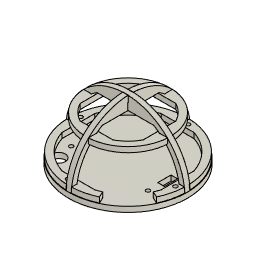
Ball prototype (Autodesk Fusion 360 design; units mm, degrees)
Autodesk Fusion 360 part; units mm, degrees
sketch "Schizzo2" plane through (0, 0, 0) normal (1, 0, 0) x (0, 1, 0)
  circle A0 centre (0, 0) radius 45 construction
  line L0 (0, -45) -> (0, -43.7069)
  line L1 (0, -43.7069) -> (0, 45)
  line L2 (0, 0) -> (44.9555, 0) construction
  line L3 (44.9555, 0) -> (44.9555, 2)
  line L4 (44.9555, 0) -> (44.9555, -2)
  line L5 (0, 0) -> (-44.9555, 0) construction
  line L6 (44.9555, 2) -> (-44.9555, 2)
  line L7 (-44.9555, 2) -> (-44.9555, 0)
  line L8 (44.9555, -2) -> (-44.9555, -2)
  line L9 (-44.9555, 0) -> (-44.9555, -2)
  line L10 (44.5982, 6) -> (44.5982, 2)
  line L11 (44.5982, 6) -> (-44.5982, 6)
  line L12 (-44.5982, 6) -> (-44.5982, 2)
  arc A1 (44.9555, 2) -> (-44.9555, 2) centre (0, 0) ccw
  arc A2 (40.9512, 2) -> (-40.9512, 2) centre (0, 0) ccw
  line L13 (2, 44.9555) -> (2, 34.9555)
  line L14 (-2, 44.9555) -> (-2, 34.9555)
  line L15 (-2, 34.9555) -> (-21.4269, 34.9555)
  line L16 (2, 34.9555) -> (21.4269, 34.9555)
  line L17 (2, 34.9555) -> (-2, 34.9555)
  line L18 (2, 39.9555) -> (-2, 39.9555)
  line L19 (1.8, 39.9555) -> (1.8, 34.9555)
  line L20 (-1.8, 39.9555) -> (-1.8, 34.9555)
  line L21 (1.8, 39.9555) -> (1.8, 44.964)
  line L22 (-1.8, 39.9555) -> (-1.8, 44.964)
  line L23 (0, 0) -> (31.8198, 31.8198) construction
  line L24 (31.8198, 31.8198) -> (-31.8198, 31.8198)
  line L25 (-31.8198, 31.8198) -> (-31.8198, 27.8198)
  line L26 (-31.8198, 27.8198) -> (31.8198, 27.8198)
  line L27 (31.8198, 27.8198) -> (31.8198, 31.8198)
  line L28 (25.8554, 31.8198) -> (25.8554, 27.8198)
  line L29 (-25.8554, 31.8198) -> (-25.8554, 27.8198)
  dimension "d3" = 90
  dimension "d5" = 4
  dimension "d6" = 4
  dimension "d9" = 10
  dimension "d10" = 4
  dimension "d11" = 4
  dimension "d18" = 0.2
  dimension "d19" = 0.2
  dimension "d39" = 45
  dimension "d40" = 4
  constraint coincident A0.centre L2.start
  constraint coincident A0 L0.start
  constraint coincident A0.centre L0
  constraint coincident A0 L1.end
  constraint coincident A0.centre L1
  constraint vertical L1
  constraint perpendicular L1 L2
  constraint coincident A0 L3.end
  constraint perpendicular L2 L3
  constraint coincident A0 L4.end
  constraint perpendicular L2 L4
  constraint perpendicular L1 L5
  constraint coincident A0 L6.end
  constraint perpendicular L3 L6
  constraint coincident A0 L8.end
  constraint perpendicular L4 L8
  constraint perpendicular L5 L7
  constraint coincident A0 L10.start
  constraint coincident L6 L10.end
  constraint perpendicular L6 L10
  constraint coincident A0 L11.end
  constraint perpendicular L10 L11
  constraint coincident L6 L12.end
  constraint perpendicular L6 L12
  constraint coincident L6 A2.end
  constraint coincident L6 A2.start
  constraint vertical L13
  constraint coincident A2 L15.end
  constraint perpendicular L14 L15
  constraint coincident A2 L16.end
  constraint perpendicular L13 L16
  constraint collinear L15 L16
  constraint coincident A0 L13.start
  constraint coincident A1 L14.start
  constraint equal L13 L14
  constraint midpoint L13 L18.start
  constraint midpoint L14 L18.end
  constraint coincident L18 L19.start
  constraint coincident L17 L19.end
  constraint perpendicular L17 L19
  constraint coincident L18 L20.start
  constraint coincident L17 L20.end
  constraint perpendicular L17 L20
  constraint coincident A0 L21.end
  constraint coincident A0 L22.end
  constraint perpendicular L18 L21
  constraint perpendicular L18 L22
  constraint coincident A1 L23.end
  constraint horizontal L24
  constraint vertical L25
  constraint horizontal L26
  constraint vertical L27
  constraint coincident A1 L24.end
  constraint coincident A2 L28.start
  constraint coincident L24 L28.start
  constraint coincident L26 L28.end
  constraint perpendicular L26 L28
  constraint coincident A2 L29.start
  constraint coincident L24 L29.start
  constraint coincident L26 L29.end
  constraint perpendicular L26 L29
  measures "d3" diameter of A0
  measures "d5" distance of L6 L8
  measures "d6" distance of L11.end L12.end
  measures "d9" distance of L13.start L13.end
  measures "d10" distance of L18.start L18.end
  measures "d11" distance of A0 A2
  measures "d18" distance of L14 L20
  measures "d19" distance of L13 L19
  measures "d39" angle of L1 L23
  measures "d40" distance of L24.end L25.end
revolve "Rivoluzione1" add sketch "Schizzo2" angle 360 about axis through (0, 0, -43.7069) along (0, 0, 1) contours L1 L6 L7 L8 L9 makes body 1
revolve "Rivoluzione2" add sketch "Schizzo2" angle 360 about axis through (0, 0, -43.7069) along (0, 0, 1) separate body contours L1 L6 L11 A2 | L6 L11 L12 A2 picked at (-13.5195, 4.6667) makes body 2
revolve "Rivoluzione3" add sketch "Schizzo2" angle 360 about axis through (0, 0, -43.7069) along (0, 0, 1) separate body contours L1 L24 L26 L29 | A2 L26 L29 | A2 L24 L25 L26 makes body 3
extrude "Estrusione1" add sketch "Schizzo2" along normal mid plane 4 separate body contours L6 L10 L11 A2 | L6 L11 L12 A2 | L11 A1 A2 L26 L27 | L11 A1 A2 L25 L26 | L6 L10 A1 | L6 L12 A1 | A2 L26 L29 | A2 L26 L28 | A2 L24 L26 L27 | A2 L24 L25 L26 | A1 A2 L13 L24 | A1 A2 L14 L24 | L1 A2 L18 L22 | L1 A2 L18 L21 | L13 L17 L18 L19 | L14 L17 L18 L20 | A2 L13 L16 | A2 L14 L15 | A1 A2 L13 L21 | A1 A2 L14 L22 | L1 A1 A2 L22 | L1 A1 A2 L21 | A2 L13 L18 L21 | A2 L14 L18 L22 makes body 4
extrude "Estrusione2" add sketch "Schizzo2" along normal mid plane 4 separate body contours L6 L10 L11 A2 | L6 L11 L12 A2 | L11 A1 A2 L26 L27 | L11 A1 A2 L25 L26 | L6 L10 A1 | L6 L12 A1 | A2 L26 L29 | A2 L26 L28 | A2 L24 L26 L27 | A2 L24 L25 L26 | L1 L17 L18 L20 | L1 L17 L18 L19 | A1 A2 L13 L24 | A1 A2 L14 L24 | L13 L17 L18 L19 | L14 L17 L18 L20 | A2 L13 L16 | A2 L14 L15 | A1 A2 L13 L21 | A1 A2 L14 L22 | A2 L13 L18 L21 | A2 L14 L18 L22 makes body 5
sketch "Schizzo3" plane through (0, 0, 6) normal (0, 0, 1) x (-1, 0, 0)
  circle A0 centre (0, 0) radius 44.5982
  circle A1 centre (0, 0) radius 35.5
  circle A2 centre (0, 0) radius 37.5
  line L0 (0, 0) -> (44.5982, 0) construction
  line L1 (40.3982, 0) -> (40.3982, -1.8)
  line L2 (40.3982, -1.8) -> (44.5619, -1.8)
  line L3 (40.3982, 0) -> (40.3982, 1.8)
  line L4 (40.3982, 1.8) -> (44.5619, 1.8)
  circle A3 centre (0, 0) radius 39.5
  line L5 (37.5, 0) -> (37.5, 12.4097)
  line L6 (37.5, 0) -> (37.5, -12.4097)
  line L7 (1.8, 40.3982) -> (1.8, 44.5619)
  line L8 (0, 40.3982) -> (1.8, 40.3982)
  line L9 (-1.8, 40.3982) -> (-1.8, 44.5619)
  line L10 (0, 40.3982) -> (-1.8, 40.3982)
  line L11 (0, 37.5) -> (12.4097, 37.5)
  line L12 (0, 37.5) -> (-12.4097, 37.5)
  line L13 (-40.3982, 1.8) -> (-44.5619, 1.8)
  line L14 (-40.3982, 0) -> (-40.3982, 1.8)
  line L15 (-40.3982, -1.8) -> (-44.5619, -1.8)
  line L16 (-40.3982, 0) -> (-40.3982, -1.8)
  line L17 (-37.5, 0) -> (-37.5, 12.4097)
  line L18 (-37.5, 0) -> (-37.5, -12.4097)
  line L19 (-1.8, -40.3982) -> (-1.8, -44.5619)
  line L20 (0, -40.3982) -> (-1.8, -40.3982)
  line L21 (1.8, -40.3982) -> (1.8, -44.5619)
  line L22 (0, -40.3982) -> (1.8, -40.3982)
  line L23 (0, -37.5) -> (-12.4097, -37.5)
  line L24 (0, -37.5) -> (12.4097, -37.5)
  circle A4 centre (40.5982, -4.8) radius 1.5
  circle A5 centre (4.8, 40.5982) radius 1.5
  circle A6 centre (-40.5982, 4.8) radius 1.5
  circle A7 centre (-4.8, -40.5982) radius 1.5
  line L25 (0, 0) -> (-31.5357, 31.5357) construction
  line L26 (0, 0) -> (-40.4197, 18.848)
  line L27 (0, 0) -> (-18.848, 40.4197)
  dimension "d22" = 71
  dimension "d23" = 2
  dimension "d26" = 4.2
  dimension "d27" = 3.6
  dimension "d28" = 4
  dimension "d30" = 360
  dimension "d33" = 3
  dimension "d34" = 3
  dimension "d35" = 0.2
  dimension "d36" = 135
  dimension "d37" = 20
  dimension "d38" = 20
  constraint concentric A0 A1
  constraint concentric A1 A2
  constraint coincident A0.centre A1.centre
  constraint coincident A0 L0.end
  constraint horizontal L0
  constraint coincident L0 L1.start
  constraint perpendicular L0 L1
  constraint coincident A0 L2.end
  constraint perpendicular L0 L3
  constraint equal L1 L3
  constraint coincident A0 L4.end
  constraint perpendicular L1 L2
  constraint perpendicular L3 L4
  constraint concentric A2 A3
  constraint coincident A2 L5.start
  constraint coincident L0 L5.start
  constraint coincident A3 L5.end
  constraint tangent A2 L5
  constraint coincident A3 L6.end
  constraint tangent A2 L6
  constraint coincident A0 L25.end
  constraint coincident A0 L26.end
  constraint coincident A0 L27.end
  measures "d22" diameter of A1
  measures "d23" distance of A1 A2
  measures "d26" distance of L0.end L1
  measures "d27" distance of L2 L4
  measures "d28" distance of A1 A3
  measures "d33" diameter of A4
  measures "d34" distance of L2 A4.centre
  measures "d35" distance of L1 A4.centre
  measures "d36" angle of L0 L25
  measures "d37" angle of L25 L26
  measures "d38" angle of L25 L27
extrude "Estrusione3" cut sketch "Schizzo3" against normal blind 4 contours A0 L1 L2 L3 L4 | A0 L7 L8 L9 L10 | A0 L19 L20 L21 L22 | A0 A3 L26 L27 | A0 L13 L14 L15 L16 | A2 A3 L26 L27 | A2 A3 L12 L27 | A2 A3 L17 L26 | A1 A2 L26 L27 | A1 A2 L26 L27 | A3 A5 | A3 A5 | A2 A3 L5 L11 | A1 L26 L27 | A1 L26 L27 | A3 A6 | A3 A6 | A2 A3 L18 L23 | A2 A3 L6 L24 | A3 A4 | A3 A4 | A3 A7 | A3 A7 bodies 2
sketch "Schizzo4" plane through (0, 0, 31.8198) normal (0, 0, 1) x (-1, 0, 0)
  circle A0 centre (0, 0) radius 31.8198
  line L0 (0, 31.8198) -> (0, -31.8198) construction
  circle A1 centre (0, 0) radius 23.8198
  circle A2 centre (0, 0) radius 26.8198
  line L1 (0, -23.8198) -> (12.3255, -23.8198)
  line L2 (0, -23.8198) -> (-12.3255, -23.8198)
  line L3 (2, -25.8554) -> (-2, -25.8554)
  line L4 (-2, -25.8554) -> (-2, -30.1174)
  line L5 (2, -30.1174) -> (2, -25.8554)
  line L6 (1.8, -31.7689) -> (1.8, -26.0554)
  line L7 (1.8, -26.0554) -> (-1.8, -26.0554)
  line L8 (-1.8, -26.0554) -> (-1.8, -31.7689)
  line L9 (26.0554, -1.8) -> (31.7689, -1.8)
  line L10 (26.0554, 1.8) -> (26.0554, -1.8)
  line L11 (31.7689, 1.8) -> (26.0554, 1.8)
  line L12 (23.8198, 0) -> (23.8198, 12.3255)
  line L13 (23.8198, 0) -> (23.8198, -12.3255)
  line L14 (1.8, 26.0554) -> (1.8, 31.7689)
  line L15 (-1.8, 26.0554) -> (1.8, 26.0554)
  line L16 (-1.8, 31.7689) -> (-1.8, 26.0554)
  line L17 (0, 23.8198) -> (-12.3255, 23.8198)
  line L18 (0, 23.8198) -> (12.3255, 23.8198)
  line L19 (-26.0554, 1.8) -> (-31.7689, 1.8)
  line L20 (-26.0554, -1.8) -> (-26.0554, 1.8)
  line L21 (-31.7689, -1.8) -> (-26.0554, -1.8)
  line L22 (-23.8198, 0) -> (-23.8198, -12.3255)
  line L23 (-23.8198, 0) -> (-23.8198, 12.3255)
  point P0 (0, 31.8198)
  dimension "d44" = 5
  dimension "d45" = 8
  dimension "d62" = 0.2
  dimension "d63" = 0.2
  dimension "d64" = 0.2
  dimension "d66" = 360
  constraint coincident P0 L0.start
  constraint coincident A0 L0.end
  constraint vertical L0
  constraint concentric A0 A1
  constraint concentric A1 A2
  constraint coincident L0 L1.start
  constraint coincident A1 L1.start
  constraint coincident A2 L1.end
  constraint tangent A1 L1
  constraint coincident A2 L2.end
  constraint tangent A1 L2
  constraint coincident A0 L6.start
  constraint parallel L5 L6
  constraint perpendicular L5 L7
  constraint coincident A0 L8.end
  constraint perpendicular L7 L8
  measures "d44" distance of A0 A2
  measures "d45" distance of A0 A1
  measures "d62" distance of L5 L6
  measures "d63" distance of L4 L8
  measures "d64" distance of L3 L7
extrude "Estrusione4" cut sketch "Schizzo4" against normal blind 4 contours A0 A2 L9 L11 | A0 A2 L14 L16 | A2 L9 L10 L11 | A0 A2 L6 L8 | A2 L14 L15 L16 | A1 A2 L12 L18 | A2 L6 L7 L8 | A1 A2 L1 L13 | A0 A2 L19 L21 | A1 | A2 L19 L20 L21 | A1 A2 L17 L23 | A1 A2 L2 L22 bodies 3
sketch "Schizzo5" plane through (0, 0, 2) normal (0, 0, 1) x (-1, 0, 0)
  circle A0 centre (0, 0) radius 44.9555
  circle A1 centre (0, 0) radius 35.5 construction
  circle A2 centre (29, 13.8789) radius 1.5
  circle A3 centre (-29, 13.8789) radius 1.5
  line L0 (0, 0) -> (0, 35.5) construction
  line L1 (-29, 13.8789) -> (0, 13.8789) construction
  line L2 (0, 13.8789) -> (29, 13.8789) construction
  line L3 (-29, 13.8789) -> (0, 0) construction
  line L4 (-29, 13.8789) -> (-32.0218, 15.325) construction
  circle A4 centre (40.5982, -4.8) radius 1.5
  circle A5 centre (-40.5982, 4.8) radius 1.5
  circle A6 centre (4.8, 40.5982) radius 1.5
  circle A7 centre (-4.8, -40.5982) radius 1.5
  line L5 (0, 0) -> (-30, 0) construction
  line L6 (0, 0) -> (30, 0) construction
  line L7 (27.5, -5) -> (32.5, -5)
  line L8 (32.5, -5) -> (32.5, 5)
  line L9 (32.5, 5) -> (27.5, 5)
  line L10 (27.5, 5) -> (27.5, -5)
  line L11 (27.5, -5) -> (32.5, 5) construction
  line L12 (32.5, -5) -> (27.5, 5) construction
  line L13 (-27.5, -5) -> (-32.5, -5)
  line L14 (-32.5, -5) -> (-32.5, 5)
  line L15 (-32.5, 5) -> (-27.5, 5)
  line L16 (-27.5, 5) -> (-27.5, -5)
  line L17 (-27.5, -5) -> (-32.5, 5) construction
  line L18 (-32.5, -5) -> (-27.5, 5) construction
  line L19 (0, 0) -> (31.7884, 31.7884) construction
  circle A8 centre (26.163, 26.163) radius 5
  point P0 (30, 0)
  point P1 (-30, 0)
  dimension "d50" = 71
  dimension "d51" = 3
  dimension "d52" = 58
  dimension "d53" = 3.35
  dimension "d56" = 10
  dimension "d57" = 5
  dimension "d58" = 60
  dimension "d59" = 45
  dimension "d60" = 10
  dimension "d61" = 37
  constraint coincident A0.centre A1.centre
  constraint coincident A1 L0.end
  constraint vertical L0
  constraint coincident A3.centre L1.start
  constraint coincident L0 L1.end
  constraint perpendicular L0 L1
  constraint coincident A2.centre L2.end
  constraint perpendicular L0 L2
  constraint equal L1 L2
  constraint coincident A1 L4.end
  constraint parallel L3 L4
  constraint equal A2 A3
  constraint perpendicular L0 L5
  constraint perpendicular L0 L6
  constraint horizontal L7
  constraint perpendicular L7 L8
  constraint parallel L7 L9
  constraint parallel L8 L10
  constraint coincident L11 P0
  constraint coincident L12 P0
  constraint coincident P0 L6.end
  constraint horizontal L13
  constraint perpendicular L13 L14
  constraint parallel L13 L15
  constraint parallel L14 L16
  constraint coincident L17 P1
  constraint coincident L18 P1
  constraint coincident P1 L5.end
  constraint equal L7 L13
  constraint equal L10 L16
  constraint equal L5 L6
  constraint coincident A0 L19.end
  constraint coincident L19 A8.centre
  measures "d50" diameter of A1
  measures "d51" diameter of A2
  measures "d52" distance of A2.centre A3.centre
  measures "d53" distance of A3.centre L4.end
  measures "d56" distance of L7.end L8.end
  measures "d57" distance of L7.start L7.end
  measures "d58" distance of P0 P1
  measures "d59" angle of L0 L19
  measures "d60" diameter of A8
  measures "d61" distance of A0.centre A8.centre
extrude "Estrusione5" cut sketch "Schizzo5" against normal blind 4 contours A2 | A3 | A4 | A5 | A6 | A7 | L7 L8 L9 L10 | L13 L14 L15 L16 | A8 bodies 1
move_body "Sposta1" bodies 4 to x (0, -1, 0) y (1, 0, 0) z (0, 0, 1) at (0, 0, 0)
equation "d = 90 mm"
equation "d3 = d"
equation "h = 4 mm"
equation "d5 = h"
equation "d6 = h"
equation "d10 = h"
equation "dPCB = 71 mm"
equation "d15 = h / 2"
equation "t = 0.2 mm"
equation "d18 = t"
equation "d19 = t"
equation "d22 = dPCB"
equation "d26 = t + 4 mm"
equation "d27 = h - 2 * t"
equation "d31 = -h"
equation "d40 = h"
equation "d48 = -h"
equation "d50 = dPCB"
equation "d52 = 55.3 mm + ( 2.7 ) * 1 mm"
equation "d53 = 2 mm + ( 2.7 / 2 ) * 1 mm"
equation "d54 = -h"
equation "d62 = t"
equation "d63 = t"
equation "d64 = t"
named bodies: "mid", "anchor", "arch1", "arch2", "support"
